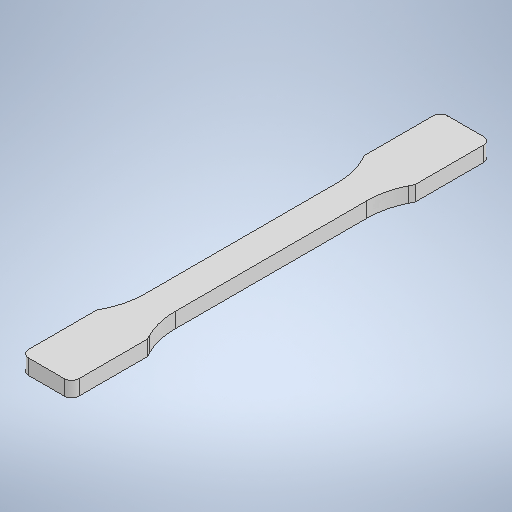
# Autodesk Inventor part: 10x5_Probestück
Saved by Autodesk Inventor 2025 (Build 290162000, 162)
## iProperties
Created: 2026-05-29
Part Number: 10x5_Probestück
Material: Generisch
Document SubType Name: Modeling
Designer: uwedo
Density: 1 g/cm^3
Appearance: Vorgabe
Author: uwedo
Autodesk Inventor part; units mm, degrees
ref_plane "YZ Plane" through (0, 0, 0) normal (1, 0, 0) x (0, 1, 0)
ref_plane "XZ Plane" through (0, 0, 0) normal (0, 1, 0) x (-1, 0, 0)
ref_plane "XY Plane" through (0, 0, 0) normal (0, 0, 1) x (1, 0, 0)
sketch "Skizze1" plane through (0, 0, 0) normal (0, 0, 1) x (1, 0, 0)
  line L0 (0, 0) -> (20, 0)
  line L1 (20, 0) -> (20, 30)
  line L2 (20, 30) -> (0, 30)
  line L3 (0, 30) -> (0, 0)
  line L4 (4, 38) -> (16, 38)
  line L5 (16, 38) -> (16, 128)
  line L6 (16, 128) -> (4, 128)
  line L7 (4, 128) -> (4, 38)
  line L8 (0, 136) -> (20, 136)
  line L9 (20, 136) -> (20, 166)
  line L10 (20, 166) -> (0, 166)
  line L11 (0, 166) -> (0, 136)
  line L12 (0, 136) -> (4, 128)
  line L13 (4, 38) -> (0, 30)
  line L14 (16, 38) -> (20, 30)
  line L15 (20, 136) -> (16, 128)
  point P0 (10, 38)
  point P1 (10, 128)
  dimension "d0" = 20
  dimension "d1" = 30
  dimension "d2" = 20
  dimension "d3" = 30
  dimension "d4" = 10
  dimension "d5" = 90
  dimension "d6" = 8
  dimension "d7" = 8
  dimension "d8" = 10
  dimension "d9" = 12
  constraints: 32 end point, 6 parallel, 3 horizontal, 3 perpendicular, 2 midpoint
  measures "d0" distance between parallel lines of L1 L3
  measures "d1" distance between parallel lines of L0 L2
  measures "d2" distance between parallel lines of L9 L11
  measures "d3" distance between parallel lines of L8 L10
  measures "d4" distance from line of L3 point (10, 38)
  measures "d5" distance between parallel lines of L4 L6
  measures "d6" distance between parallel lines of L6 L8
  measures "d7" distance between parallel lines of L2 L4
  measures "d8" distance from line of point (10, 128) L11
  measures "d9" distance between parallel lines of L5 L7
extrude "Extrusion1" add sketch "Skizze1" along normal blind 6
fillet "Rundung1" radius 3 4 edges at (20, 0, 3) (0, 0, 3) (20, 166, 3) (0, 166, 3)
fillet "Rundung2" radius 30 4 edges at (4, 128, 3) (4, 38, 3) (16, 38, 3) (16, 128, 3)
